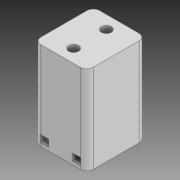
# Autodesk Inventor part: IR Headtracker riser
Saved by Autodesk Inventor 2020 (Build 240168000, 168)
## iProperties
Created: 2021-03-06
Part Number: IR Headtracker riser
Material: Generic
Document SubType Name: Modeling
Designer: Arsenio
Density: 1 g/cm^3
Appearance: Default
Author: Arsenio
Autodesk Inventor part; units mm, degrees
ref_plane "YZ Plane" through (0, 0, 0) normal (1, 0, 0) x (0, 1, 0)
ref_plane "XZ Plane" through (0, 0, 0) normal (0, 1, 0) x (-1, 0, 0)
ref_plane "XY Plane" through (0, 0, 0) normal (0, 0, 1) x (1, 0, 0)
sketch "Sketch1" plane through (0, 0, 0) normal (0, 1, 0) x (-1, 0, 0)
  circle A0 centre (0, -12.557) radius 1.5
  circle A1 centre (0, -22.557) radius 1.5
  arc A2 (-14.605, -9.6379) -> (-15.8103, -6.9952) centre (-18.105, -9.6379) ccw
  line L0 (-14.605, -29.4809) -> (-14.605, -9.6379)
  line L1 (13.605, -29.4809) -> (-14.605, -29.4809)
  line L2 (13.605, -12.0588) -> (13.605, -29.4809)
  arc A3 (14.5665, -9.2788) -> (13.605, -12.0588) centre (18.105, -12.0588) ccw
  line L3 (0, -22.557) -> (0, -12.557)
  line L4 (-8, -8.557) -> (8, -8.557)
  line L5 (8, -8.557) -> (8, -26.557)
  line L6 (8, -26.557) -> (-8, -26.557)
  line L7 (-8, -26.557) -> (-8, -8.557)
  line L8 (-8, -8.557) -> (8, -26.557) construction
  line L9 (8, -8.557) -> (-8, -26.557) construction
  point P0 (0, -17.557)
  dimension "d0" = 3
  dimension "d1" = 3
  dimension "d2" = 10
  dimension "d3" = 16
  dimension "d4" = 18
  constraints: 20 end point, 4 centre point, 4 point on circle, 3 midpoint, 2 parallel, 1 horizontal, 1 perpendicular, 1 vertical
  measures "d0" diameter of A0
  measures "d1" diameter of A1
  measures "d2" distance of L3.start L3.end
  measures "d3" distance of L5.end L6.end
  measures "d4" distance of L4.end L5.end
extrude "Extrusion1" add sketch "Sketch1" along normal blind 27
extrude "Extrusion2" add sketch "Sketch1" along normal blind 17 contours A0 | A1
fillet "Fillet1" radius 2 4 edges at (-8, 13.5, -8.557) (8, 13.5, -8.557) (-8, 13.5, -26.557) (8, 13.5, -26.557)
sketch "Sketch2" plane through (-6, 0, -8.557) normal (0, 0, 1) x (1, 0, 0)
  line L0 (-0.15, 3.1878) -> (2.35, 3.1878)
  line L1 (2.35, 3.1878) -> (2.35, 1.0878)
  line L2 (2.35, 1.0878) -> (-0.15, 1.0878)
  line L3 (-0.15, 1.0878) -> (-0.15, 3.1878)
  line L4 (-0.15, 3.1878) -> (2.35, 1.0878) construction
  line L5 (2.35, 3.1878) -> (-0.15, 1.0878) construction
  line L6 (9.6689, 3.1878) -> (12.1689, 3.1878)
  line L7 (12.1689, 3.1878) -> (12.1689, 1.0878)
  line L8 (12.1689, 1.0878) -> (9.6689, 1.0878)
  line L9 (9.6689, 1.0878) -> (9.6689, 3.1878)
  line L10 (9.6689, 3.1878) -> (12.1689, 1.0878) construction
  line L11 (12.1689, 3.1878) -> (9.6689, 1.0878) construction
  line L12 (-0.15, 2.1378) -> (12.15, 2.1378) construction
  line L13 (6, 0) -> (6, 2.1378)
  point P0 (1.1, 2.1378)
  point P1 (10.9189, 2.1378)
  point P2 (12.1689, 2.1378)
  dimension "d10" = 2.5
  dimension "d11" = 2.1
  dimension "d12" = 2.5
  dimension "d13" = 2.1
  dimension "d14" = 12.3
  constraints: 28 end point, 7 midpoint, 4 parallel, 3 horizontal, 2 perpendicular, 1 vertical
  measures "d10" distance of L1.end L2.end
  measures "d11" distance of L0.end L1.end
  measures "d12" distance of L7.end L8.end
  measures "d13" distance of L6.end L7.end
  measures "d14" distance of L12.start L12.end
extrude "Extrusion3" cut sketch "Sketch2" against normal blind 19.5
body "Solid1"
